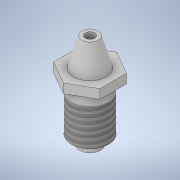
# Autodesk Inventor part: ZKE-Term-Solid
Saved by Autodesk Inventor 2021 (Build 250183000, 183)
## iProperties
Created: 2020-06-09
Part Number: ZKE-Term-Solid
Material: Generic
Document SubType Name: Modeling
Designer: lucas
Density: 1 g/cm^3
Appearance: Default
Project: 4Wire
Author: lucas
Revision Number: ZKE_SOLID
Autodesk Inventor part; units mm, degrees
ref_plane "YZ Plane" through (0, 0, 0) normal (1, 0, 0) x (0, 1, 0)
sketch "Sketch1" plane through (0, 0, 0) normal (0, 1, 0) x (-1, 0, 0)
  line L0 (0, 5.7735) -> (5, 2.8868)
  line L1 (5, 2.8868) -> (5, -2.8868)
  line L2 (5, -2.8868) -> (0, -5.7735)
  line L3 (0, -5.7735) -> (-5, -2.8868)
  line L4 (-5, -2.8868) -> (-5, 2.8868)
  line L5 (-5, 2.8868) -> (0, 5.7735)
  point P0 (0, 0)
  dimension "d24" = 10
  constraints: 12 end point, 13 other
  measures "d24" distance between parallel lines of L5 L2
extrude "Extrusion1" add sketch "Sketch1" along normal blind 2
sketch "Sketch2" plane through (0, 2, 0) normal (0, 1, 0) x (1, 0, 0)
  circle A0 centre (0, 0) radius 3.5
  dimension "d2" = 7
  constraints: 1 centre point
  measures "d2" diameter of A0
ref_plane "Work Plane1" through (0, 8, 0) normal (0, 1, 0) x (1, 0, 0)
sketch "Sketch3" plane through (0, 8, 0) normal (0, 1, 0) x (1, 0, 0)
  circle A0 centre (0, 0) radius 1.75
  dimension "d4" = 3.5
  constraints: 1 centre point
  measures "d4" diameter of A0
loft "Loft1" add profiles "Sketch2", "Sketch3"
sketch "Sketch4" plane through (0, 0, 0) normal (0, -1, 0) x (1, 0, 0)
  circle A0 centre (0, 0) radius 4
  dimension "d9" = 8
  constraints: 1 centre point
  measures "d9" diameter of A0
extrude "Extrusion2" add sketch "Sketch4" along normal blind 10.4
thread "Thread1" size "M8x1.25" class "6g" standard "ANSI Metric M Profile" length 8 offset 2.4
sketch "Sketch5" plane through (0, 8, 0) normal (0, 1, 0) x (1, 0, 0)
  circle A0 centre (0, 0) radius 1
  dimension "d14" = 2
  constraints: 1 centre point
  measures "d14" diameter of A0
ref_plane "Work Plane2" through (0, -12.4, 0) normal (0, -1, 0) x (1, 0, 0)
sketch "Sketch6" plane through (0, -12.4, 0) normal (0, -1, 0) x (1, 0, 0)
  circle A0 centre (0, 0) radius 2.25
  dimension "d16" = 4.5
  constraints: 1 centre point
  measures "d16" diameter of A0
sketch "Sketch7" plane through (0, -10.4, 0) normal (0, -1, 0) x (1, 0, 0)
  circle A0 centre (0, 0) radius 3.25
  dimension "d17" = 6.5
  constraints: 1 centre point
  measures "d17" diameter of A0
loft "Loft2" add profiles "Sketch7", "Sketch6"
extrude "Extrusion3" cut sketch "Sketch5" against normal up to surface (20.4 mm away)
body "Solid1"
